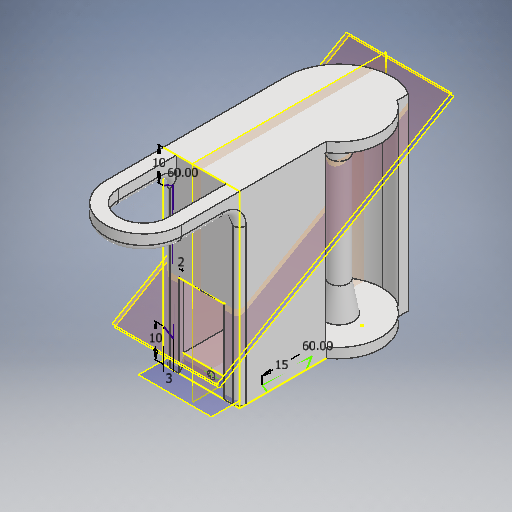
# Autodesk Inventor part: body
Saved by Autodesk Inventor 2025.2 (Build 292293000, 293)
## iProperties
Created: 2025-03-09
Part Number: body
Material: Generic
Document SubType Name: Modeling
Designer: Alex
Density: 1 g/cm^3
Appearance: Default
Author: Alex
Autodesk Inventor part; units mm, degrees
ref_plane "YZ Plane" through (0, 0, 0) normal (1, 0, 0) x (0, 1, 0)
ref_plane "XZ Plane" through (0, 0, 0) normal (0, 1, 0) x (-1, 0, 0)
ref_plane "XY Plane" through (0, 0, 0) normal (0, 0, 1) x (1, 0, 0)
sketch "Sketch1" plane through (0, 0, 0) normal (1, 0, 0) x (0, 1, 0)
  line L0 (0, 0) -> (0, -9.15) construction
  line L1 (0, -9.15) -> (9.0687, -2.8) construction
  line L2 (9.0687, -2.8) -> (9.0687, 0) construction
  line L3 (0, -9.15) -> (0, -29.4542) construction
  line L4 (0, 0) -> (49.8191, 0) construction
  line L5 (9.0687, 0) -> (0, 0)
  line L6 (9.0687, -2.8) -> (25.35, -2.8)
  line L7 (25.35, -2.8) -> (25.35, 0)
  line L8 (25.35, 0) -> (9.0687, 0)
  line L9 (9.0687, -2.8) -> (0, -4.3991)
  line L10 (0, 0) -> (0, -4.3991)
  dimension "d1" = 125
  dimension "d2" = 5.6
  dimension "d3" = 9.15
  dimension "d5" = 9.0687
  dimension "d6" = 25.35
  dimension "d8" = 80
  constraints: 22 end point, 3 collinear, 2 horizontal, 2 point on line, 2 vertical, 1 parallel, 1 perpendicular
  measures "d1" angle of L3 L1
  measures "d2" diameter of L1.end L4
  measures "d3" distance of L0.start L0.end
  measures "d5" distance of L0.start L2.end
  measures "d6" distance between parallel lines of L3 L7
  measures "d8" angle of L0 L9
revolve "Revolution1" add sketch "Sketch1" angle 360 about axis through (0, 0, 0) along (0, 1, 0)
sketch "Sketch2" plane through (0, 0, 0) normal (0, -1, 0) x (1, 0, 0)
  line L0 (6.9, -13.1) -> (-16.1, -13.1) construction
  line L1 (-16.1, -13.1) -> (-16.1, 36.9)
  line L2 (-16.1, 36.9) -> (6.9, 36.9)
  line L3 (6.9, 36.9) -> (6.9, -13.1) construction
  circle A0 centre (0, 0) radius 12.5 construction
  circle A1 centre (0, 0) radius 13 construction
  line L4 (6.9, -13.1) -> (6.9, -11.0177) construction
  line L5 (6.9, 36.9) -> (6.9, 11.0177)
  line L6 (0, -13.1) -> (0, -13) construction
  line L7 (3.9, 12.4012) -> (3.9, 33.9)
  line L8 (3.9, 33.9) -> (-13.1, 33.9)
  line L9 (-13.1, 33.9) -> (-13.1, 0)
  arc A2 (6.9, 11.0177) -> (3.9, 12.4012) centre (0, 0) ccw
  arc A3 (-13.1, 0) -> (0, -13.1) centre (0, 0) ccw
  line L10 (0, -13.1) -> (0, -16.1) construction
  line L11 (-13.1, 0) -> (-13, 0) construction
  circle A4 centre (0, 0) radius 2.8 projected
  line L12 (0, 0) -> (-13, 0) construction
  arc A5 (0, -13.1) -> (6.9, -11.0177) centre (0.1762, -1.2107) ccw
  line L13 (-13.1, 0) -> (-16.1, 0) construction
  arc A6 (-16.1, 0) -> (0, -16.1) centre (0, 0) ccw
  line L14 (6.9, -11.0177) -> (6.9, -14.0177)
  arc A7 (0, -16.1) -> (6.9, -14.0177) centre (0, -3.6267) ccw
  dimension "d9" = 25
  dimension "d10" = 0.5
  dimension "d11" = 3
  dimension "d12" = 3
  dimension "d13" = 3
  dimension "d15" = 3
  dimension "d16" = 23
  dimension "d18" = 0.1
  dimension "d19" = 0.1
  dimension "d22" = 3
  dimension "d23" = 11.8906
  dimension "d24" = 50
  constraints: 30 end point, 15 point on circle, 7 centre point, 5 perpendicular, 4 point on line, 4 tangent, 3 horizontal, 3 vertical, 2 parallel, 1 coincident, 1 concentric
  measures "d9" diameter of A0
  measures "d10" radial gap between concentric circles of A0 A1
  measures "d11" distance between parallel lines of L1 L9
  measures "d12" distance between parallel lines of L8 L2
  measures "d13" distance between parallel lines of L7 L3
  measures "d15" distance of L6.start L10.end
  measures "d16" distance of L0.start L0.end
  measures "d18" distance of L9.end L11.end
  measures "d19" distance of L6.start L6.end
  measures "d22" distance of L4.end L14.end
  measures "d23" radius of A5
  measures "d24" distance of L0.end L1.end
extrude "Extrusion1" add sketch "Sketch2" against normal up to surface (25.35 mm away) contours L1 L2 L5 A2 L7 L8 L9 A3 A5 L14 A7 A6
sketch "Sketch3" plane through (0, 0, 0) normal (0, -1, 0) x (1, 0, 0)
  line L0 (6.9, 11.0177) -> (6.9, 36.9) projected
  line L1 (6.9, 36.9) -> (-16.1, 36.9) projected
  line L2 (-16.1, 36.9) -> (-16.1, 0) projected
  arc A0 (-16.1, 0) -> (0, -16.1) centre (0, 0) ccw projected
  arc A1 (0, -16.1) -> (6.9, -14.0177) centre (0, -3.6267) ccw projected
  line L3 (6.9, -14.0177) -> (6.9, -11.0177) projected
  arc A2 (0, -13.1) -> (6.9, -11.0177) centre (0.1762, -1.2107) ccw construction
  line L4 (6.9, 11.0177) -> (6.9, -11.0177) construction
  arc A3 (6.9, -10.4177) -> (6.9, 10.4177) centre (-0.0081, 0) ccw construction
  arc A4 (6.9, -10.6569) -> (6.9, 10.6569) centre (-0.0081, 0) ccw
  line L5 (6.9, 0) -> (12.6919, 0) construction
  line L6 (6.9, -10.6569) -> (6.9, -11.0177)
  line L7 (6.9, 11.0177) -> (6.9, 10.6569)
  point P0 (0, 0)
  dimension "d29" = 12.5
  dimension "d30" = 0.2
  dimension "d31" = 0.6
  constraints: 8 end point, 5 point on circle, 4 point on line, 2 centre point, 1 collinear, 1 horizontal, 1 midpoint, 1 vertical
  measures "d29" radius of A3
  measures "d30" radial gap between concentric circles of A3 A4
  measures "d31" distance of L3.end A3.start
extrude "Extrusion2" add sketch "Sketch3" along normal blind 3
mirror "Mirror1" about plane through (0, 25.35, 0) normal (0, 1, 0) of "Extrusion1", "Extrusion2", "Revolution1"
sketch "Sketch4" plane through (0, -3, 0) normal (0, -1, 0) x (1, 0, 0)
  line L0 (3.9, 33.9) -> (3.9, 12.4012) projected
  line L1 (-13.1, 33.9) -> (3.9, 33.9) projected
  arc A0 (6.9, 11.0177) -> (3.9, 12.4012) centre (0, 0) ccw projected
  line L2 (3.9, 15.4012) -> (6.9, 17.1506)
  line L3 (6.9, 17.1506) -> (6.9, 32.1506)
  line L4 (6.9, 10.6569) -> (6.9, 36.9) construction
  line L5 (6.9, 32.1506) -> (3.9, 33.9)
  line L6 (6.9, 36.9) -> (-16.1, 36.9) projected
  line L7 (-4.6, 36.9) -> (-4.6, -15.4289) construction
  arc A1 (-16.1, 0) -> (0, -16.1) centre (0, 0) ccw projected
  line L8 (-13.1, 15.4012) -> (-16.1, 17.1506)
  line L9 (-16.1, 17.1506) -> (-16.1, 32.1506)
  line L10 (-16.1, 32.1506) -> (-13.1, 33.9)
  line L11 (-13.1, 33.9) -> (-13.1, 15.4012)
  line L12 (-13.1, 0) -> (-13.1, 33.9) projected
  line L13 (-13.1, 33.9) -> (3.9, 33.9) projected
  line L14 (-13.1, 33.9) -> (-11.3679, 36.9)
  line L15 (3.9, 33.9) -> (2.1679, 36.9)
  point P0 (0, 0)
  dimension "d33" = 3
  dimension "d35" = 15
  dimension "d42" = 60
  constraints: 20 end point, 4 point on line, 4 symmetric about line, 2 collinear, 2 equal length, 1 midpoint, 1 point on circle, 1 vertical
  measures "d33" distance of L0.end L2.start
  measures "d35" distance of L2.end L3.end
  measures "d42" angle of L1 L14
sketch "Sketch5" plane through (-16.1, -3, 36.9) normal (0, 0, 1) x (1, 0, 0)
  line L0 (0, 0) -> (0, 56.7) projected
  line L1 (23, 0) -> (0, 0) projected
  line L2 (23, 56.7) -> (23, 0) projected
  line L3 (23, 56.7) -> (0, 56.7) projected
  line L4 (0, 10) -> (3, 8.2679)
  line L5 (3, 8.2679) -> (3, 48.4321)
  line L6 (3, 48.4321) -> (0, 46.7)
  point P0 (16.1, 3)
  dimension "d36" = 3
  dimension "d37" = 60
  dimension "d38" = 10
  dimension "d39" = 10
  constraints: 6 end point, 2 point on line, 1 equal length, 1 vertical
  measures "d36" distance from line of L5 L4.start
  measures "d37" angle of L5 L6
  measures "d38" distance of L0.start L4.start
  measures "d39" distance of L0.end L6.end
sketch "Sketch6" plane through (6.9, -3, 10.6569) normal (1, 0, 0) x (0, 0, -1)
  line L0 (0, 0) -> (-26.2431, 0) projected
  line L1 (-6.0222, 0) -> (-4.4798, 2.6716)
  line L2 (-4.4798, 2.6716) -> (-19.4798, 2.6716)
  line L3 (-19.4798, 2.6716) -> (-17.841, 0.058)
  point P0 (10.6569, 3)
  dimension "d40" = 60
  dimension "d41" = 15
  constraints: 6 end point, 1 equal length, 1 horizontal, 1 point on line
  measures "d40" angle of L2 L1
  measures "d41" distance of L1.end L2.end
extrude "Extrusion3" cut sketch "Sketch4" against normal blind 25 contours L1 L14 L6 L15
sketch "Sketch7" plane through (-13.1, 0, 33.9) normal (0, 0, 1) x (1, 0, 0)
  line L0 (0, 22) -> (1.7321, 22) projected
  line L1 (15.2679, 22) -> (17, 22) projected
  line L2 (0, 22) -> (17, 22)
  line L3 (17, 22) -> (17, 24)
  line L4 (17, 24) -> (0, 24)
  line L5 (0, 24) -> (0, 22)
  point P0 (13.1, 0)
  dimension "d45" = 2
  constraints: 8 end point, 2 perpendicular, 1 horizontal, 1 parallel
  measures "d45" distance of L4.end L0.start
ref_plane "Work Plane1" through (-13.1, 22, 33.9) normal (0, -0.8660254, -0.5) x (1, 0, 0)
ref_plane "Work Plane2" through (-10.35, 22, 36.9) normal (0, 0.8660254, 0.5) x (1, 0, 0)
sketch "Sketch8" plane through (-10.35, 22, 36.9) normal (0, 0.8660254, 0.5) x (1, 0, 0)
  point P0 (10.35, 20.9563)
ref_plane "Work Plane3" through (-4.6, -3, 10.6569) normal (1, 0, 0) x (0, 0, -1)
sketch "Sketch9" plane through (0, 22, 0) normal (0, -1, 0) x (1, 0, 0)
  line L0 (-11.3679, 36.9) -> (2.1679, 36.9) projected
  line L1 (-13.1, 33.9) -> (-11.3679, 36.9) projected
  line L2 (3.9, 33.9) -> (-13.1, 33.9) projected
  line L3 (2.1679, 36.9) -> (3.9, 33.9) projected
  point P0 (0, 0)
sketch "Sketch10" plane through (-10.35, 22, 36.9) normal (0, 0.8660254, 0.5) x (1, 0, 0)
  line L0 (12.5179, 0) -> (14.25, 2.5981) projected
  line L1 (-1.0179, 0) -> (12.5179, 0) projected
  line L2 (12.5179, 0) -> (-1.0179, 0)
  line L3 (-1.0179, 0) -> (-1.0179, 4.37)
  line L4 (-1.0179, 4.37) -> (12.5179, 4.37)
  line L5 (12.5179, 4.37) -> (12.5179, 0)
  point P0 (10.35, 20.9563)
  constraints: 8 end point, 3 perpendicular, 1 collinear
sketch "Sketch11" plane through (-13.1, 0, 33.9) normal (0, 0, 1) x (1, 0, 0)
  line L0 (0, 0) -> (17, 0) construction
  line L1 (0, -3) -> (0, 0) construction
  line L2 (17, -3) -> (0, -3) construction
  line L3 (17, -3) -> (17, 0) construction
  line L4 (13.1, 0) -> (0, 0) projected
  line L5 (8.5, 0) -> (8.5, -3) construction
  point P0 (8.5, -1.5)
  constraints: 2 end point, 2 midpoint, 1 point on line
ref_plane "Work Plane4" through (-4.6, -1.5, 33.9) normal (0, -1, 0) x (1, 0, 0)
sketch "Sketch12" plane through (-4.6, -1.5, 33.9) normal (0, -1, 0) x (1, 0, 0)
  line L0 (-8.5, 0) -> (8.5, 0) projected
  line L1 (0, 0) -> (0, 0.85) construction
  arc A0 (0.85, 0) -> (0, 0.85) centre (0, 0) ccw construction
  line L2 (8.5, 0) -> (-8.5, 0) projected
  line L3 (0, 0) -> (0, -0.85)
  arc A1 (0, -0.85) -> (0.85, 0) centre (0, 0) ccw
  point P0 (4.6, -33.9)
  dimension "d48" = 0.85
  dimension "d49" = 0.85
  constraints: 4 end point, 4 point on circle, 3 line through centre, 2 centre point, 2 vertical, 1 midpoint, 1 point on line
  measures "d48" distance of L1.start L1.end
  measures "d49" distance of L3.start L3.end
revolve "Revolution2" cut sketch "Sketch12" angle 360 about axis through (-4.6, -1.5, 33.9) along (0, 0, -1)
fillet "Fillet1" radius 0.3 1 edges at (-5.45, -1.5, 33.9)
sketch "Sketch14" plane through (-16.1, 53.7, 36.9) normal (0, 1, 0) x (1, 0, 0)
  line L0 (23, 0) -> (0, 0) projected
  arc A0 (0, -17.5) -> (23, -17.5) centre (11.5, -17.5) ccw
  arc A1 (4, -17.5) -> (19, -17.5) centre (11.5, -17.5) ccw
  line L1 (23, -17.5) -> (23, 0)
  line L2 (19, -17.5) -> (19, 0)
  line L3 (4, -17.5) -> (4, 0)
  line L4 (0, -17.5) -> (0, 0)
  point P0 (16.1, 36.9)
  point P1 (11.5, 0)
  point P2 (11.5, -25)
  dimension "d54" = 25
  dimension "d55" = 4
  constraints: 8 end point, 5 point on circle, 4 tangent, 3 perpendicular, 2 centre point, 2 point on line, 1 concentric, 1 midpoint, 1 vertical
  measures "d54" distance of point (11.5, 0) point (11.5, -25)
  measures "d55" distance between parallel lines of L1 L2
extrude "Extrusion4" add sketch "Sketch14" against normal blind 5 contours L1 A0 L4 L0 L3 A1 L2
fillet "Fillet2" radius 5 2 edges at (4.9, 48.7, 36.9) (-14.1, 48.7, 36.9)
fillet "Fillet3" radius 2 5 edges at (2.9, 48.7, 48.15) (2.9, 47.2355, 38.3645) (-12.1, 48.7, 48.15) (-12.1, 47.2355, 38.3645) (-4.6, 48.7, 61.9)
fillet "Fillet4" radius 2 7 edges at (-16.1, 48.7, 48.15) (-16.1, 47.2355, 38.3645) (-16.1, 20.35, 36.9) (6.9, 48.7, 48.15) (6.9, 47.2355, 38.3645) (6.9, 20.35, 36.9) (-4.6, 48.7, 65.9)
body "Solid1"
